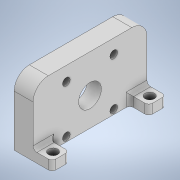
# Autodesk Inventor part: Soporte_motor_aluminio
Saved by Autodesk Inventor 2022 (Build 260153000, 153)
## iProperties
Created: 2022-12-06
Part Number: Soporte_motor_aluminio
Material: Genérico
Document SubType Name: Modeling
Designer: Usuario
Density: 1 g/cm^3
Appearance: Valor por defecto
Author: Usuario
Autodesk Inventor part; units mm, degrees
ref_plane "YZ Plane" through (0, 0, 0) normal (1, 0, 0) x (0, 1, 0)
ref_plane "XZ Plane" through (0, 0, 0) normal (0, 1, 0) x (-1, 0, 0)
ref_plane "XY Plane" through (0, 0, 0) normal (0, 0, 1) x (1, 0, 0)
sketch "Boceto1" plane through (0, 0, 0) normal (1, 0, 0) x (0, 1, 0)
  line L0 (0, 0) -> (35, 0)
  line L1 (35, 0) -> (35, -60)
  line L2 (35, -60) -> (0, -60)
  line L3 (0, -60) -> (0, 0)
  circle A0 centre (15, -30) radius 6
  circle A1 centre (27.5, -17.5) radius 2
  circle A2 centre (27.5, -42.5) radius 2
  circle A3 centre (2.5, -42.5) radius 2
  circle A4 centre (2.5, -17.5) radius 2
  dimension "d0" = 60
  dimension "d1" = 35
  dimension "d2" = 20
  dimension "d3" = 30
  dimension "d4" = 12
  dimension "d5" = 12.5
  dimension "d6" = 12.5
  dimension "d7" = 12.5
  dimension "d8" = 12.5
  dimension "d9" = 12.5
  dimension "d10" = 12.5
  dimension "d11" = 12.5
  dimension "d12" = 12.5
  dimension "d13" = 4
  dimension "d14" = 4
  dimension "d15" = 4
  dimension "d16" = 4
  constraints: 8 end point, 5 centre point, 2 parallel, 1 horizontal, 1 perpendicular
  measures "d0" distance between parallel lines of L2 L0
  measures "d1" distance between parallel lines of L1 L3
  measures "d2" distance from line of A0.centre L1
  measures "d3" distance from line of A0.centre L2
  measures "d4" diameter of A0
  measures "d5" horizontal distance of A3.centre A0.centre
  measures "d6" horizontal distance of A4.centre A0.centre
  measures "d7" horizontal distance of A1.centre A0.centre
  measures "d8" horizontal distance of A2.centre A0.centre
  measures "d9" horizontal distance of A2.centre A0.centre
  measures "d10" horizontal distance of A1.centre A0.centre
  measures "d11" horizontal distance of A4.centre A0.centre
  measures "d12" horizontal distance of A3.centre A0.centre
  measures "d13" diameter of A1
  measures "d14" diameter of A2
  measures "d15" diameter of A3
  measures "d16" diameter of A4
extrude "Extrusión1" add sketch "Boceto1" along normal blind 10
sketch "Boceto3" plane through (10, 0, 0) normal (1, 0, 0) x (0, 0, -1)
  circle A0 centre (30, 15) radius 6 projected
  circle A1 centre (30, 15) radius 22
  line L0 (0, 35) -> (0, 0) projected
  line L1 (0, 0) -> (9, 0)
  line L2 (9, 0) -> (9, 5)
  line L3 (9, 5) -> (0, 5)
  line L4 (0, 5) -> (0, 0)
  line L5 (0, 0) -> (60, 0) projected
  line L6 (60, 0) -> (51, 0)
  line L7 (51, 0) -> (51, 5)
  line L8 (51, 5) -> (60, 5)
  line L9 (60, 5) -> (60, 0)
  point P0 (0, 5)
  dimension "d19" = 44
  dimension "d20" = 9
  dimension "d21" = 5
  dimension "d22" = 9
  dimension "d23" = 5
  constraints: 16 end point, 4 parallel, 2 horizontal, 2 perpendicular, 1 centre point, 1 coincident
  measures "d19" diameter of A1
  measures "d20" distance between parallel lines of L2 L0
  measures "d21" distance between parallel lines of L3 L1
  measures "d22" distance between parallel lines of L9 L7
  measures "d23" distance between parallel lines of L8 L5
extrude "Extrusión2" add sketch "Boceto3" along normal blind 10 contours L7 L8 L9 L5 | L1 L0 L3 L2
fillet "Empalme1" radius 2 4 edges at (10, 5, -4.5) (10, 5, -55.5) (10, 2.5, -9) (10, 2.5, -51)
sketch "Boceto4" plane through (20, 5, 0) normal (0, 1, 0) x (1, 0, 0)
  line L0 (-8, 9) -> (0, 9) projected
  line L1 (-8, 0) -> (0, 0) projected
  line L2 (-8, 60) -> (0, 60) projected
  line L3 (0, 9) -> (0, 0) projected
  line L4 (0, 60) -> (0, 51) projected
  point P0 (-20, 0)
  point P1 (-4, 4.5)
  point P2 (-4, 55.5)
  dimension "d27" = 4.5
  dimension "d28" = 9
  dimension "d29" = 4.5
  dimension "d30" = 4
  dimension "d31" = 4
  measures "d27" distance from line of point (-4, 4.5) L0
  measures "d28" distance between parallel lines of L0 L1
  measures "d29" distance from line of point (-4, 55.5) L2
  measures "d30" distance from line of point (-4, 4.5) L3
  measures "d31" distance from line of point (-4, 55.5) L4
hole "Agujero1" at (16, 5, -4.5) at (16, 5, -55.5) direction (0, -1, 0) diameter 5 end through all
fillet "Empalme2" radius 8 2 edges at (5, 35, 0) (5, 35, -60)
sketch "Boceto5" plane through (0, 0, 0) normal (-1, 0, 0) x (0, 0, 1)
  circle A0 centre (-30, 15) radius 6 projected
  circle A1 centre (-30, 15) radius 13
  point P0 (0, 0)
  dimension "d40" = 26
  constraints: 1 centre point, 1 coincident
  measures "d40" diameter of A1
extrude "Extrusión3" cut sketch "Boceto5" against normal blind 2.6
fillet "Empalme3" radius 2 4 edges at (20, 2.5, 0) (20, 2.5, -9) (20, 2.5, -51) (20, 2.5, -60)
equation "\"d3\" = 0.5 * d0"
equation "\"d6\" = d5"
equation "\"d7\" = d5"
equation "\"d8\" = d5"
equation "\"d9\" = d5"
equation "\"d10\" = d5"
equation "\"d11\" = d5"
equation "\"d12\" = d5"
equation "\"d14\" = d13"
equation "\"d15\" = d13"
equation "\"d16\" = d13"
equation "\"d22\" = d20"
equation "\"d27\" = 0.5 * d28"
equation "\"d29\" = d27"
equation "\"d31\" = d30"
